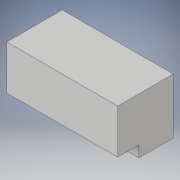
# Autodesk Inventor part: orthographic4
Saved by Autodesk Inventor 2017 (Build 210142000, 142)
## iProperties
Created: 2018-12-03
Part Number: orthographic4
Material: Generic
Document SubType Name: Modeling
Designer: qthuynh
Density: 1 g/cm^3
Appearance: Default
Author: qthuynh
Autodesk Inventor part; units mm, degrees
ref_plane "YZ Plane" through (0, 0, 0) normal (1, 0, 0) x (0, 1, 0)
ref_plane "XZ Plane" through (0, 0, 0) normal (0, 1, 0) x (-1, 0, 0)
ref_plane "XY Plane" through (0, 0, 0) normal (0, 0, 1) x (1, 0, 0)
sketch "Sketch1" plane through (0, 0, 0) normal (0, 0, 1) x (1, 0, 0)
  line L0 (0, 0) -> (203.2, 0)
  line L1 (203.2, 0) -> (203.2, 101.6)
  line L2 (203.2, 101.6) -> (0, 101.6)
  line L3 (0, 101.6) -> (0, 0)
  dimension "d0" = 203.2
  dimension "d1" = 101.6
  constraints: 8 end point, 2 parallel, 1 horizontal, 1 perpendicular
  measures "d0" distance of L2.end L1.end
  measures "d1" distance of L1.end L0.end
extrude "Extrusion1" add sketch "Sketch1" along normal blind 101.6
sketch "Sketch2" plane through (203.2, 0, 0) normal (1, 0, 0) x (0, 0, -1)
  line L0 (0, 0) -> (-101.6, 0) projected
  line L1 (-101.6, 0) -> (-62.738, 0)
  line L2 (-62.738, 0) -> (-101.6, 0)
  line L3 (-62.738, 0) -> (-62.738, 20.574)
  line L4 (-62.738, 20.574) -> (-101.6, 20.574)
  line L5 (-101.6, 0) -> (-101.6, 101.6) projected
  line L6 (-101.6, 20.574) -> (-101.6, 0)
  dimension "d4" = 38.862
  dimension "d5" = 20.574
  constraints: 10 end point, 2 collinear, 1 perpendicular, 1 point on line, 1 vertical
  measures "d4" distance of L0.end L1.end
  measures "d5" distance of L1.end L3.end
extrude "Extrusion2" cut sketch "Sketch2" against normal blind 203.2
body "Solid1"
